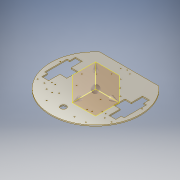
# Autodesk Inventor part: BottomPlate
Saved by Autodesk Inventor 2019 (Build 230136000, 136)
## iProperties
Created: 2020-02-28
Part Number: BottomPlate
Material: Generic
Document SubType Name: Modeling
Designer: james
Mass: 617.778 g
Surface Area: 2655.15 cm^2
Volume: 617.778 cm^3
Density: 1 g/cm^3
Appearance: Titanium
Author: james
Autodesk Inventor part; units mm, degrees
ref_plane "YZ Plane" through (0, 0, 0) normal (1, 0, 0) x (0, 1, 0)
ref_plane "XZ Plane" through (0, 0, 0) normal (0, 1, 0) x (-1, 0, 0)
ref_plane "XY Plane" through (0, 0, 0) normal (0, 0, 1) x (1, 0, 0)
sketch "Sketch1" plane through (0, 0, 0) normal (0, 1, 0) x (-1, 0, 0)
  circle A0 centre (0, 0) radius 203.2
  dimension "d0" = 406.4
  constraints: 1 centre point, 1 coincident
  measures "d0" diameter of A0
extrude "Extrusion1" add sketch "Sketch1" along normal blind 4.7625
sketch "Sketch2" plane through (0, 4.7625, 0) normal (0, 1, 0) x (1, 0, 0)
  line L0 (-165.1, -76.2) -> (-139.7, -76.2)
  line L1 (-139.7, -76.2) -> (-139.7, 76.2)
  line L2 (-139.7, 76.2) -> (-165.1, 76.2)
  line L3 (-165.1, 76.2) -> (-165.1, -76.2)
  line L4 (139.7, 76.2) -> (165.1, 76.2)
  line L5 (165.1, 76.2) -> (165.1, -76.2)
  line L6 (165.1, -76.2) -> (139.7, -76.2)
  line L7 (139.7, -76.2) -> (139.7, 76.2)
  point P0 (0, 0)
  dimension "d3" = 25.4
  dimension "d4" = 25.4
  dimension "d5" = 0
  dimension "d6" = 0
  dimension "d7" = 152.4
  dimension "d8" = 76.2
  dimension "d9" = 139.7
  dimension "d10" = 139.7
  constraints: 16 end point, 4 parallel, 2 horizontal, 2 perpendicular
  measures "d3" distance of L5.end L6.end
  measures "d4" distance of L0.start L0.end
  measures "d5" distance between parallel lines of L6 L0
  measures "d6" distance between parallel lines of L4 L2
  measures "d7" distance of L4.end L5.end
  measures "d8" distance from line of point (0, 0) L6
  measures "d9" distance from line of L1 point (0, 0)
  measures "d10" distance from line of L7 point (0, 0)
extrude "Extrusion2" cut sketch "Sketch2" against normal blind 28.575
sketch "Sketch4" plane through (0, 0, 0) normal (0, -1, 0) x (1, 0, 0)
  line L0 (-136.525, 76.2) -> (-167.64, 76.2)
  line L1 (-167.64, 76.2) -> (-167.64, -76.2)
  line L2 (-167.64, -76.2) -> (-136.525, -76.2)
  line L3 (-136.525, -76.2) -> (-136.525, 76.2)
  line L4 (-139.7, -76.2) -> (-165.1, -76.2) projected
  line L5 (-165.1, 76.2) -> (-139.7, 76.2) projected
  line L6 (-165.1, -76.2) -> (-165.1, 76.2) projected
  line L7 (-139.7, 76.2) -> (-139.7, -76.2) projected
  point P0 (0, 0)
  dimension "d24" = 0
  dimension "d25" = 0
  dimension "d26" = 2.54
  dimension "d27" = 3.175
  constraints: 8 end point, 2 parallel, 1 horizontal, 1 perpendicular
  measures "d24" distance between parallel lines of L2 L4
  measures "d25" distance between parallel lines of L5 L0
  measures "d26" distance between parallel lines of L6 L1
  measures "d27" distance between parallel lines of L7 L3
extrude "Extrusion3" cut sketch "Sketch4" against normal blind 11.1125 contours L3 L2 L7 L0 | L6 L2 L1 L0
sketch "Sketch8" plane through (0, 4.7625, 0) normal (0, 1, 0) x (1, 0, 0)
  line L0 (-249.9736, 258.2829) -> (238.9858, 258.2829)
  line L1 (238.9858, 258.2829) -> (238.9858, 152.4)
  line L2 (238.9858, 152.4) -> (-249.9736, 152.4)
  line L3 (-249.9736, 152.4) -> (-249.9736, 258.2829)
  point P0 (0, 0)
  dimension "d80" = 152.4
  constraints: 8 end point, 2 parallel, 1 horizontal, 1 perpendicular
  measures "d80" distance from line of point (0, 0) L2
extrude "Extrusion4" cut sketch "Sketch8" against normal blind 100.0125
sketch "Sketch9" plane through (0, 4.7625, 0) normal (0, 1, 0) x (1, 0, 0)
  line L0 (-142.7514, 25.4) -> (-104.775, 25.4)
  line L1 (-104.775, 25.4) -> (-104.775, -25.4)
  line L2 (-104.775, -25.4) -> (-142.7514, -25.4)
  line L3 (-142.7514, -25.4) -> (-142.7514, 25.4)
  line L4 (-136.525, 76.2) -> (-136.525, -76.2) projected
  line L5 (-167.64, 76.2) -> (-136.525, 76.2) projected
  point P0 (0, 0)
  dimension "d83" = 50.8
  dimension "d84" = 31.75
  dimension "d85" = 50.8
  constraints: 8 end point, 2 parallel, 1 horizontal, 1 perpendicular
  measures "d83" distance of L0.end L1.end
  measures "d84" distance between parallel lines of L4 L1
  measures "d85" distance between parallel lines of L5 L0
extrude "Extrusion5" cut sketch "Sketch9" against normal blind 9.525
sketch "Sketch10" plane through (0, 4.7625, 0) normal (0, 1, 0) x (1, 0, 0)
  line L0 (149.2619, 25.4) -> (107.95, 25.4)
  line L1 (107.95, 25.4) -> (107.95, -25.4)
  line L2 (107.95, -25.4) -> (149.2619, -25.4)
  line L3 (149.2619, -25.4) -> (149.2619, 25.4)
  line L4 (-104.775, -25.4) -> (-136.525, -25.4) projected
  line L5 (-136.525, 25.4) -> (-104.775, 25.4) projected
  line L6 (139.7, -76.2) -> (139.7, 76.2) projected
  point P0 (0, 0)
  dimension "d97" = 0
  dimension "d98" = 0
  dimension "d99" = 31.75
  constraints: 8 end point, 2 parallel, 1 horizontal, 1 perpendicular
  measures "d97" distance between parallel lines of L4 L2
  measures "d98" distance between parallel lines of L5 L0
  measures "d99" distance between parallel lines of L1 L6
extrude "Extrusion6" cut sketch "Sketch10" against normal blind 25.4
sketch "Sketch11" plane through (0, 4.7625, 0) normal (0, 1, 0) x (1, 0, 0)
  line L0 (-136.525, -76.2) -> (-167.64, -76.2) projected
  line L1 (-136.525, -25.4) -> (-136.525, -76.2) projected
  line L2 (139.7, -76.2) -> (139.7, -25.4) projected
  point P0 (0, 0)
  point P1 (-121.92, -76.2)
  point P2 (-106.68, -76.2)
  point P3 (106.68, -76.2)
  point P4 (121.92, -76.2)
  dimension "d102" = 0
  dimension "d103" = 0
  dimension "d104" = 0
  dimension "d106" = 15.24
  dimension "d107" = 15.24
  dimension "d221" = 106.68
  dimension "d222" = 106.68
  dimension "d223" = 76.2
  measures "d102" vertical distance of point (106.68, -76.2) point (121.92, -76.2)
  measures "d103" vertical distance of point (-106.68, -76.2) point (106.68, -76.2)
  measures "d104" vertical distance of point (-106.68, -76.2) point (-121.92, -76.2)
  measures "d106" distance of point (-106.68, -76.2) point (-121.92, -76.2)
  measures "d107" distance of point (121.92, -76.2) point (106.68, -76.2)
  measures "d221" horizontal distance of point (-106.68, -76.2) point (0, 0)
  measures "d222" horizontal distance of point (0, 0) point (106.68, -76.2)
  measures "d223" vertical distance of point (0, 0) point (-106.68, -76.2)
hole "Hole5" at (-121.92, 4.7625, 76.2) at (-106.68, 4.7625, 76.2) at (106.68, 4.7625, 76.2) at (121.92, 4.7625, 76.2) direction (0, -1, 0) diameter 4.4958 end through all clearance for "Hex Machine Screw" size "#8" standard "Ansi Unified Screw Threads"
sketch "Sketch12" plane through (0, 4.7625, 0) normal (0, 1, 0) x (1, 0, 0)
  circle A0 centre (106.68, -76.2) radius 2.2479 projected
  circle A1 centre (-106.68, -76.2) radius 2.2479 projected
  point P0 (0, 0)
  point P1 (-87.63, 25.4)
  point P2 (87.63, 25.4)
  point P3 (-185.42, 25.4)
  point P4 (185.42, 25.4)
  dimension "d117" = 101.6
  dimension "d118" = 19.05
  dimension "d119" = 19.05
  dimension "d120" = 101.6
  dimension "d121" = 0
  dimension "d122" = 0
  dimension "d123" = 97.79
  dimension "d124" = 97.79
  measures "d117" vertical distance of A1.centre point (-87.63, 25.4)
  measures "d118" horizontal distance of A1.centre point (-87.63, 25.4)
  measures "d119" horizontal distance of A0.centre point (87.63, 25.4)
  measures "d120" vertical distance of A0.centre point (87.63, 25.4)
  measures "d121" vertical distance of point (185.42, 25.4) point (87.63, 25.4)
  measures "d122" vertical distance of point (-87.63, 25.4) point (-185.42, 25.4)
  measures "d123" distance of point (-87.63, 25.4) point (-185.42, 25.4)
  measures "d124" distance of point (87.63, 25.4) point (185.42, 25.4)
hole "Hole6" at (-87.63, 4.7625, -25.4) at (87.63, 4.7625, -25.4) at (-185.42, 4.7625, -25.4) at (185.42, 4.7625, -25.4) direction (0, -1, 0) diameter 4.4958 end through all clearance for "Hex Machine Screw" size "#8" standard "Ansi Unified Screw Threads"
sketch "Sketch13" plane through (0, 4.7625, 0) normal (0, 1, 0) x (1, 0, 0)
  line L0 (136.525, -76.2) -> (167.64, -76.2)
  line L1 (167.64, -76.2) -> (167.64, 76.2)
  line L2 (167.64, 76.2) -> (136.525, 76.2)
  line L3 (136.525, 76.2) -> (136.525, -76.2)
  line L4 (139.7, 76.2) -> (165.1, 76.2) projected
  line L5 (165.1, -76.2) -> (139.7, -76.2) projected
  line L6 (139.7, -76.2) -> (139.7, -25.4) projected
  line L7 (165.1, 76.2) -> (165.1, -76.2) projected
  point P0 (0, 0)
  dimension "d132" = 0
  dimension "d133" = 0
  dimension "d134" = 3.175
  dimension "d135" = 2.54
  constraints: 8 end point, 2 parallel, 1 horizontal, 1 perpendicular
  measures "d132" distance between parallel lines of L4 L2
  measures "d133" distance between parallel lines of L5 L0
  measures "d134" distance between parallel lines of L6 L3
  measures "d135" distance between parallel lines of L7 L1
extrude "Extrusion7" cut sketch "Sketch13" against normal blind 14.2875
sketch "Sketch14" plane through (0, 4.7625, 0) normal (0, 1, 0) x (1, 0, 0)
  point P0 (0, 0)
  point P1 (-63.5, -101.6)
  point P2 (63.5, -101.6)
  point P3 (63.5, -158.75)
  point P4 (-63.5, -158.75)
  dimension "d138" = 0
  dimension "d139" = 0
  dimension "d140" = 0
  dimension "d141" = 0
  dimension "d142" = 57.15
  dimension "d143" = 127
  dimension "d144" = 63.5
  dimension "d145" = 101.6
  measures "d138" vertical distance of point (63.5, -101.6) point (-63.5, -101.6)
  measures "d139" vertical distance of point (63.5, -158.75) point (-63.5, -158.75)
  measures "d140" horizontal distance of point (63.5, -101.6) point (63.5, -158.75)
  measures "d141" horizontal distance of point (-63.5, -101.6) point (-63.5, -158.75)
  measures "d142" distance of point (-63.5, -158.75) point (-63.5, -101.6)
  measures "d143" distance of point (63.5, -158.75) point (-63.5, -158.75)
  measures "d144" horizontal distance of point (0, 0) point (63.5, -158.75)
  measures "d145" vertical distance of point (-63.5, -101.6) point (0, 0)
hole "Hole7" at (-63.5, 4.7625, 101.6) at (63.5, 4.7625, 101.6) at (63.5, 4.7625, 158.75) at (-63.5, 4.7625, 158.75) direction (0, -1, 0) diameter 4.4958 end through all clearance for "Hex Machine Screw" size "#8" standard "Ansi Unified Screw Threads"
sketch "Sketch15" plane through (0, 4.7625, 0) normal (0, 1, 0) x (1, 0, 0)
  point P0 (0, 0)
  point P1 (82.55, -97.79)
  point P2 (110.744, -154.813)
  dimension "d153" = 97.79
  dimension "d154" = 82.55
  dimension "d155" = 57.023
  dimension "d156" = 28.194
  measures "d153" vertical distance of point (82.55, -97.79) point (0, 0)
  measures "d154" horizontal distance of point (0, 0) point (82.55, -97.79)
  measures "d155" vertical distance of point (110.744, -154.813) point (82.55, -97.79)
  measures "d156" horizontal distance of point (82.55, -97.79) point (110.744, -154.813)
hole "Hole8" at (82.55, 4.7625, 97.79) at (110.744, 4.7625, 154.813) direction (0, -1, 0) diameter 4.4958 end through all clearance for "Hex Machine Screw" size "#8" standard "Ansi Unified Screw Threads"
sketch "Sketch16" plane through (0, 4.7625, 0) normal (0, 1, 0) x (1, 0, 0)
  circle A0 centre (0, 113.9) radius 29.5
  line L0 (134.4042, 152.4) -> (-134.4042, 152.4) projected
  line L1 (0, 113.9) -> (-31.602, 145.502)
  line L2 (0, 113.9) -> (0, 152.4)
  line L3 (0, 113.9) -> (25.919, 139.819)
  line L4 (0, 113.9) -> (-24.7208, 89.1792)
  line L5 (0, 113.9) -> (28.4179, 85.4821)
  point P0 (0, 0)
  point P1 (0, 143.4)
  point P2 (-20.8597, 134.7597)
  point P3 (20.8597, 134.7597)
  point P4 (-20.8597, 93.0403)
  point P5 (20.8597, 93.0403)
  dimension "d164" = 0
  dimension "d165" = 38.5
  dimension "d166" = 59
  dimension "d167" = 45
  dimension "d168" = 45
  dimension "d169" = 90
  dimension "d170" = 90
  constraints: 10 end point, 5 point on circle, 5 point on line, 1 centre point, 1 midpoint, 1 vertical
  measures "d164" horizontal distance of point (0, 0) L1.start
  measures "d165" distance from line of L1.start L0
  measures "d166" diameter of A0
  measures "d167" angle of L1 L2
  measures "d168" angle of L3 L2
  measures "d169" angle of L5 L3
  measures "d170" angle of L4 L5
hole "Hole9" at (0, 4.7625, -143.4) at (-20.8597, 4.7625, -134.7597) at (20.8597, 4.7625, -134.7597) at (-20.8597, 4.7625, -93.0403) at (20.8597, 4.7625, -93.0403) direction (0, -1, 0) diameter 3.4036 depth 25.4 tip angle 118 clearance for "Flat Head Machine Screw" size "M3" standard "Ansi Metric M Profile"
sketch "Sketch17" plane through (0, 4.7625, 0) normal (0, 1, 0) x (1, 0, 0)
  point P0 (0, 0)
  point P1 (-54.61, 57.15)
  point P2 (54.61, 57.15)
  point P3 (54.61, -31.75)
  point P4 (-54.61, -31.75)
  dimension "d178" = 0
  dimension "d179" = 0
  dimension "d180" = 0
  dimension "d181" = 0
  dimension "d182" = 109.22
  dimension "d183" = 88.9
  dimension "d184" = 54.61
  dimension "d185" = 57.15
  measures "d178" vertical distance of point (-54.61, -31.75) point (54.61, -31.75)
  measures "d179" horizontal distance of point (54.61, 57.15) point (54.61, -31.75)
  measures "d180" horizontal distance of point (-54.61, -31.75) point (-54.61, 57.15)
  measures "d181" vertical distance of point (54.61, 57.15) point (-54.61, 57.15)
  measures "d182" distance of point (-54.61, 57.15) point (54.61, 57.15)
  measures "d183" distance of point (-54.61, -31.75) point (-54.61, 57.15)
  measures "d184" horizontal distance of point (-54.61, 57.15) point (0, 0)
  measures "d185" vertical distance of point (0, 0) point (54.61, 57.15)
hole "Hole10" at (-54.61, 4.7625, -57.15) at (54.61, 4.7625, -57.15) at (54.61, 4.7625, 31.75) at (-54.61, 4.7625, 31.75) direction (0, -1, 0) diameter 4.4958 end through all clearance for "Flat Head Machine Screw (82)" size "#8" standard "Ansi Unified Screw Threads"
sketch "Sketch18" plane through (0, 4.7625, 0) normal (0, 1, 0) x (1, 0, 0)
  point P0 (0, 0)
  point P1 (-82.55, -114.3)
  point P2 (-107.95, -114.3)
  dimension "d193" = 0
  dimension "d194" = 82.55
  dimension "d195" = 114.3
  dimension "d196" = 25.4
  measures "d193" vertical distance of point (-107.95, -114.3) point (-82.55, -114.3)
  measures "d194" horizontal distance of point (-82.55, -114.3) point (0, 0)
  measures "d195" vertical distance of point (0, 0) point (-82.55, -114.3)
  measures "d196" distance of point (-107.95, -114.3) point (-82.55, -114.3)
hole "Hole11" at (-82.55, 4.7625, 114.3) at (-107.95, 4.7625, 114.3) direction (0, -1, 0) diameter 4.4958 end through all clearance for "Flat Head Machine Screw (82)" size "#8" standard "Ansi Unified Screw Threads"
sketch "Sketch19" plane through (0, 4.7625, 0) normal (0, 1, 0) x (1, 0, 0)
  line L0 (167.64, 76.2) -> (167.64, -76.2) projected
  line L1 (136.525, -76.2) -> (136.525, -25.4) projected
  line L2 (-167.64, -76.2) -> (-167.64, 76.2) projected
  line L3 (-136.525, -25.4) -> (-136.525, -76.2) projected
  point P0 (0, 0)
  point P1 (-167.64, -95.25)
  point P2 (-136.525, -95.25)
  point P3 (136.525, -95.25)
  point P4 (167.64, -95.25)
  dimension "d204" = 0
  dimension "d205" = 0
  dimension "d206" = 0
  dimension "d207" = 19.05
  dimension "d208" = 0
  dimension "d209" = 0
  dimension "d210" = 0
  dimension "d211" = 19.05
  measures "d204" distance from line of point (167.64, -95.25) L0
  measures "d205" distance from line of point (136.525, -95.25) L1
  measures "d206" vertical distance of point (167.64, -95.25) point (136.525, -95.25)
  measures "d207" distance of point (167.64, -95.25) L0.end
  measures "d208" vertical distance of point (-167.64, -95.25) point (-136.525, -95.25)
  measures "d209" distance from line of point (-167.64, -95.25) L2
  measures "d210" distance from line of L3 point (-136.525, -95.25)
  measures "d211" distance of L2.start point (-167.64, -95.25)
hole "Hole12" at (-167.64, 4.7625, 95.25) at (-136.525, 4.7625, 95.25) at (136.525, 4.7625, 95.25) at (167.64, 4.7625, 95.25) direction (0, -1, 0) diameter 4.4958 end through all clearance for "Flat Head Machine Screw (82)" size "#8" standard "Ansi Unified Screw Threads"
sketch "Sketch20" plane through (0, 4.7625, 0) normal (0, 1, 0) x (1, 0, 0)
  line L0 (-180.34, 50.8) -> (-167.64, 50.8)
  line L1 (-167.64, 50.8) -> (-167.64, -50.8)
  line L2 (-167.64, -50.8) -> (-180.34, -50.8)
  line L3 (-180.34, -50.8) -> (-180.34, 50.8)
  line L4 (180.34, 50.8) -> (167.64, 50.8)
  line L5 (167.64, 50.8) -> (167.64, -50.8)
  line L6 (167.64, -50.8) -> (180.34, -50.8)
  line L7 (180.34, -50.8) -> (180.34, 50.8)
  line L8 (-167.64, -76.2) -> (-167.64, 76.2) projected
  line L9 (167.64, 76.2) -> (167.64, -76.2) projected
  line L10 (-167.64, 76.2) -> (-136.525, 76.2) projected
  line L11 (-136.525, -76.2) -> (-167.64, -76.2) projected
  point P0 (0, 0)
  dimension "d224" = 0
  dimension "d225" = 0
  dimension "d226" = 0
  dimension "d227" = 12.7
  dimension "d228" = 12.7
  dimension "d229" = 25.4
  dimension "d230" = 25.4
  constraints: 16 end point, 4 parallel, 2 horizontal, 2 perpendicular, 1 point on line
  measures "d224" distance between parallel lines of L6 L2
  measures "d225" distance between parallel lines of L8 L1
  measures "d226" distance between parallel lines of L9 L5
  measures "d227" distance between parallel lines of L5 L7
  measures "d228" distance between parallel lines of L1 L3
  measures "d229" distance between parallel lines of L10 L0
  measures "d230" distance between parallel lines of L11 L2
extrude "Extrusion8" cut sketch "Sketch20" against normal blind 25.4
sketch "Sketch21" plane through (0, 4.7625, 0) normal (0, 1, 0) x (1, 0, 0)
  circle A0 centre (0, -146.05) radius 12.7
  line L0 (-104.775, 25.4) -> (-104.775, -25.4) projected
  line L1 (-136.525, -76.2) -> (-167.64, -76.2) projected
  point P0 (0, 0)
  dimension "d233" = 104.775
  dimension "d234" = 69.85
  dimension "d235" = 25.4
  constraints: 1 centre point
  measures "d233" distance from line of A0.centre L0
  measures "d234" distance from line of A0.centre L1
  measures "d235" diameter of A0
extrude "Extrusion9" cut sketch "Sketch21" against normal blind 25.4
body "Solid1"
